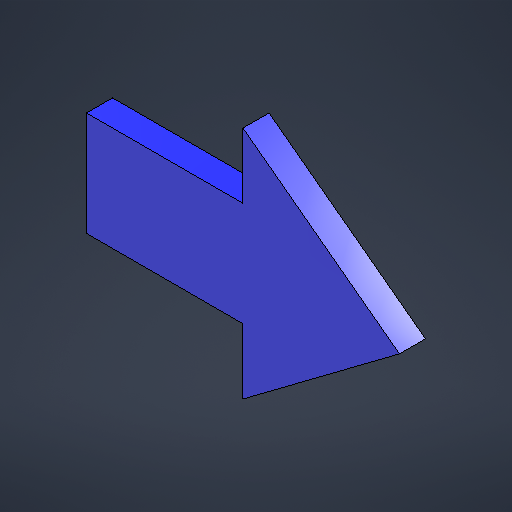
# Autodesk Inventor part: AirFlow
Saved by Autodesk Inventor 2026 (Build 300175050, 175E)
## iProperties
Project: 12345
Reference: REF01
Module: M01
Created: 2022-12-02
Part Number: AirFlow
Material: Generic
Document SubType Name: Modeling
Designer: bl
Density: 1 g/cm^3
Appearance: Blue - Wall Paint - Glossy
Checked By: Alex Rosier
Tag: ZZZ0000-8904
Author: bl
Revision Number: 1.1
Autodesk Inventor part; units mm, degrees
ref_plane "YZ Plane" through (0, 0, 0) normal (1, 0, 0) x (0, 1, 0)
ref_plane "XZ Plane" through (0, 0, 0) normal (0, 1, 0) x (-1, 0, 0)
ref_plane "XY Plane" through (0, 0, 0) normal (0, 0, 1) x (1, 0, 0)
sketch "Sketch1" plane through (0, 0, 0) normal (0, 0, 1) x (1, 0, 0)
  line L0 (-152.4, -101.6) -> (152.4, -101.6)
  line L1 (152.4, -101.6) -> (152.4, 101.6)
  line L2 (152.4, 101.6) -> (-152.4, 101.6)
  line L3 (-152.4, 101.6) -> (-152.4, -101.6)
  line L4 (-152.4, -101.6) -> (152.4, 101.6) construction
  line L5 (152.4, -101.6) -> (-152.4, 101.6) construction
  line L6 (152.4, 101.6) -> (152.4, 228.6)
  line L7 (152.4, 228.6) -> (457.2, 0)
  line L8 (457.2, 0) -> (152.4, -228.6)
  line L9 (152.4, -228.6) -> (152.4, -101.6)
  point P0 (0, 0)
  dimension "d0" = 304.8
  dimension "d1" = 203.2
  dimension "d2" = 304.8
  dimension "d3" = 457.2
  constraints: 20 end point, 5 equal length, 2 midpoint, 1 horizontal, 1 perpendicular, 1 point on line, 1 vertical
  measures "d0" distance of L2.end L1.end
  measures "d1" distance of L1.end L0.end
  measures "d2" horizontal distance of L7.end L8.end
  measures "d3" distance of L8.end L6.end
extrude "Extrusion1" add sketch "Sketch1" along normal mid plane 50.8
body "Solid1"
